Autodesk Fusion 360 part; units mm, degrees
(part 2 of 2)
sketch "Sketch2" plane through (0, 0, 38) normal (0, 0, 1) x (-1, 0, 0)
  line L0 (0, 0) -> (-42.4, 0)
  line L1 (-42.4, 0) -> (-42.4, -38.4)
  line L2 (-42.4, -38.4) -> (0, -38.4)
  line L3 (0, -38.4) -> (0, 0)
  line L4 (-42.4, -38.4) -> (0, 0) construction
  line L5 (0, -38.4) -> (-42.4, 0) construction
  line L6 (-29.6, -10.8) -> (-12.8, -10.8)
  line L7 (-12.8, -10.8) -> (-12.8, -27.6)
  line L8 (-12.8, -27.6) -> (-29.6, -27.6)
  line L9 (-29.6, -27.6) -> (-29.6, -10.8)
  line L10 (-29.6, -10.8) -> (-12.8, -27.6) construction
  line L11 (-12.8, -10.8) -> (-29.6, -27.6) construction
  point P0 (-21.2, -19.2)
  dimension "d12" = 16.8
  dimension "d13" = 16.8
  constraint coincident L1.end L2.start
  constraint coincident L0.start L3.end
  constraint coincident L2.end L3.start
  constraint coincident L0.end L1.start
  constraint perpendicular L6 L7
  constraint parallel L6 L8
  constraint parallel L7 L9
  constraint horizontal L6
  constraint coincident L10 P0
  constraint coincident L11 P0
  constraint midpoint L4 P0
  measures "d12" distance of L6.end L7.end
  measures "d13" distance of L7.end L8.end
extrude "Extrude2" add sketch "Sketch2" along normal blind 60 contours L6 L7 L8 L9
chamfer "Chamfer1" distance 1 angle 45 4 edges at (21.2, 10.8, 98) (29.6, 19.2, 98) (12.8, 19.2, 98) (21.2, 27.6, 98)
sketch "Sketch3" plane through (0, 0, 0) normal (-1, 0, 0) x (0, -1, 0)
  line L0 (0, 0) -> (0, 38)
  line L1 (0, 38) -> (-38.4, 38)
  line L2 (-38.4, 38) -> (-38.4, 0)
  line L3 (-38.4, 0) -> (0, 0)
  line L4 (-38.4, 0) -> (0, 0)
  line L5 (0, 0) -> (0, 22.4)
  line L6 (0, 22.4) -> (-38.4, 22.4)
  line L7 (-38.4, 22.4) -> (-38.4, 0)
  line L8 (-38.4, 22.4) -> (0, 0) construction
  line L9 (0, 22.4) -> (-38.4, 0) construction
  circle A0 centre (-19.2, 11.2) radius 6
  dimension "d18" = 22.4
  dimension "d19" = 12
  constraint horizontal L4
  constraint vertical L5
  constraint horizontal L6
  constraint vertical L7
  constraint coincident L2.end L3.start
  constraint midpoint L9 A0.centre
  measures "d18" distance of L2.end L6.end
  measures "d19" diameter of A0
extrude "Extrude3" cut sketch "Sketch3" against normal up to surface (6 mm away) contours A0
sketch "Sketch4" plane through (42.4, 0, 0) normal (1, 0, 0) x (0, 1, 0)
  line L0 (0, 38) -> (0, 0)
  line L1 (0, 0) -> (38.4, 0)
  line L2 (38.4, 0) -> (38.4, 38)
  line L3 (38.4, 38) -> (0, 38)
  circle A0 centre (19.2, 11.2) radius 6
  circle A1 centre (19.2, 11.2) radius 7
  dimension "d22" = 1
extrude "Extrude4" cut sketch "Sketch4" against normal up to surface (6 mm away) contours A0 | A1
thread "Thread1" "ISO Metric profile 12.0 M12x1.75 6H" major diameter 12.2265 minor diameter 10.2735 pitch 1.75 angle 60 modelled right hand crest width 0.4769 on face at (4, 13.2075, 10.9009) crest through (0.4375, 14.0633, 11.2)
fillet "Fillet1" radius 2 8 edges at (21.2, 0, 38) (0, 19.2, 38) (21.2, 38.4, 38) (42.4, 19.2, 38) (42.4, 38.4, 19) (42.4, 0, 19) (0, 0, 19) (0, 38.4, 19)
chamfer "Chamfer2" distance 1.5 angle 45 4 edges at (16.75, 0, 26.2) (25.65, 0, 26.2) (16.75, 38.4, 26.2) (25.65, 38.4, 26.2)
equation "d8 = 8 mm + 7.6 mm"
equation "d30 = 38.40 mm + 2 mm + 2 mm"
